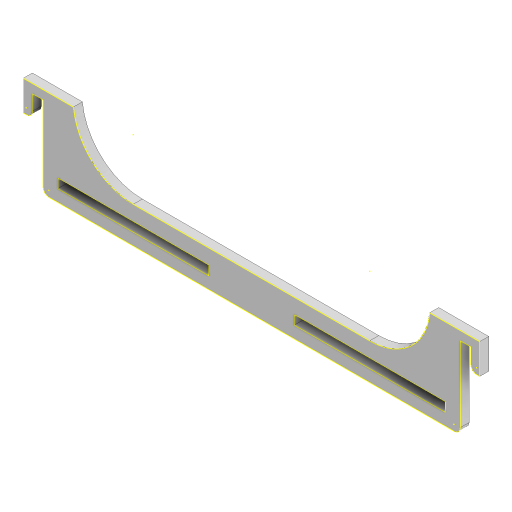
# Autodesk Inventor part: side
Saved by Autodesk Inventor 2023 (Build 270158000, 158)
## iProperties
Created: 2022-05-18
Part Number: side
Material: Generic
Document SubType Name: Modeling
Designer: Thomas
Density: 1 g/cm^3
Appearance: Default
Author: Thomas
Autodesk Inventor part; units mm, degrees
ref_plane "YZ Plane" through (0, 0, 0) normal (1, 0, 0) x (0, 1, 0)
ref_plane "XZ Plane" through (0, 0, 0) normal (0, 1, 0) x (-1, 0, 0)
ref_plane "XY Plane" through (0, 0, 0) normal (0, 0, 1) x (1, 0, 0)
sketch "Sketch1" plane through (0, 0, 0) normal (0, 0, 1) x (1, 0, 0)
  line L0 (0, 0) -> (138.5, 0)
  line L1 (138.5, 0) -> (138.5, -28)
  line L2 (136.5, -30) -> (2, -30)
  line L3 (0, -28) -> (0, 0)
  line L4 (0, 0) -> (-3.5, 0)
  line L5 (-3.5, 0) -> (-3.5, -3)
  line L6 (-3.5, -3) -> (0, -3)
  line L7 (0, -3) -> (0, 0)
  line L8 (-3.5, 0) -> (-6.5, 0)
  line L9 (-6.5, 0) -> (-6.5, -10)
  line L10 (-6.5, -10) -> (-5.5, -10)
  line L11 (-3.5, -8) -> (-3.5, 0)
  line L12 (138.5, -3) -> (142, -3)
  line L13 (142, -3) -> (142, 0)
  line L14 (142, 0) -> (138.5, 0)
  line L15 (138.5, 0) -> (138.5, -3)
  line L16 (142, 0) -> (145, 0)
  line L17 (145, 0) -> (145, -10)
  line L18 (145, -10) -> (144, -10)
  line L19 (142, -8) -> (142, 0)
  arc A0 (-5.5, -10) -> (-3.5, -8) centre (-5.5, -8) ccw
  arc A1 (142, -8) -> (144, -10) centre (144, -8) ccw
  line L20 (5, -23) -> (55, -23)
  line L21 (55, -23) -> (55, -26)
  line L22 (55, -26) -> (5, -26)
  line L23 (5, -26) -> (5, -23)
  line L24 (83.5, -23) -> (133.5, -23)
  line L25 (133.5, -23) -> (133.5, -26)
  line L26 (133.5, -26) -> (83.5, -26)
  line L27 (83.5, -26) -> (83.5, -23)
  arc A2 (0, -28) -> (2, -30) centre (2, -28) ccw
  arc A3 (136.5, -30) -> (138.5, -28) centre (136.5, -28) ccw
  point P0 (138.5, -30)
  point P1 (0, -30)
  point P2 (-3.5, -10)
  point P3 (142, -10)
  dimension "d0" = 138.5
  dimension "d1" = 30
  dimension "d2" = 3.5
  dimension "d3" = 3
  dimension "d4" = 3
  dimension "d5" = 10
  dimension "d6" = 3.5
  dimension "d7" = 3
  dimension "d8" = 3
  dimension "d9" = 10
  dimension "d10" = 2
  dimension "d11" = 3
  dimension "d12" = 20
  dimension "d13" = 5
  dimension "d14" = 50
  dimension "d15" = 3
  dimension "d16" = 5
  dimension "d17" = 50
  dimension "d18" = 2
  constraints: 56 end point, 14 parallel, 9 point on line, 8 point on circle, 8 tangent, 7 horizontal, 7 perpendicular, 4 centre point, 2 collinear, 2 equal radius
  measures "d0" distance of point (138.5, -30) point (0, -30)
  measures "d1" distance of L0.end point (138.5, -30)
  measures "d2" distance of L6.end L5.end
  measures "d3" distance of L5.end L4.end
  measures "d4" distance of point (-3.5, -10) L9.end
  measures "d5" distance of L9.end L8.end
  measures "d6" distance of L14.end L13.end
  measures "d7" distance of L13.end L12.end
  measures "d8" distance of L17.end point (142, -10)
  measures "d9" distance of L16.end L17.end
  measures "d10" radius of A0
  measures "d11" distance of L22.end L20.start
  measures "d12" distance between parallel lines of L6 L20
  measures "d13" distance between parallel lines of L3 L23
  measures "d14" distance of L20.start L20.end
  measures "d15" distance of L24.end L25.end
  measures "d16" distance between parallel lines of L1 L25
  measures "d17" distance of L24.start L24.end
  measures "d18" radius of A2
extrude "Extrusion1" add sketch "Sketch1" along normal blind 3
sketch "Sketch2" plane through (0, 0, 3) normal (0, 0, 1) x (1, 0, 0)
  line L0 (145, 0) -> (-6.5, 0) projected
  line L1 (10, 0) -> (128.5, 0)
  line L2 (128.5, 0) -> (128.5, 2)
  line L3 (108.5, -18) -> (30, -18)
  line L4 (10, 2) -> (10, 0)
  line L5 (5, -23) -> (55, -23) projected
  line L6 (0, -3) -> (0, -28) projected
  line L7 (138.5, -28) -> (138.5, -3) projected
  arc A0 (10, 2) -> (30, -18) centre (30, 2) ccw
  arc A1 (108.5, -18) -> (128.5, 2) centre (108.5, 2) ccw
  point P0 (0, 0)
  point P1 (128.3997, 0)
  point P2 (10.1003, 0)
  dimension "d21" = 5
  dimension "d22" = 10
  dimension "d23" = 10
  dimension "d24" = 20
  constraints: 8 end point, 4 point on circle, 4 tangent, 2 centre point, 2 parallel, 1 equal radius, 1 horizontal, 1 perpendicular, 1 point on line
  measures "d21" distance between parallel lines of L3 L5
  measures "d22" distance between parallel lines of L4 L6
  measures "d23" distance between parallel lines of L7 L2
  measures "d24" radius of A0
extrude "Extrusion2" cut sketch "Sketch2" against normal blind 10 contours A1 L3 A0 L0
sketch "Sketch3" plane through (0, 0, 3) normal (0, 0, 1) x (1, 0, 0)
  arc A0 (10.1003, 0) -> (30, -18) centre (30, 2) ccw projected
  line L0 (10.1003, 0) -> (-6.5, 0) projected
  line L1 (-6.5, 0) -> (-6.5, -10) projected
  line L2 (-6.5, -10) -> (-5.5, -10) projected
  arc A1 (-5.5, -10) -> (-3.5, -8) centre (-5.5, -8) ccw projected
  line L3 (-3.5, -8) -> (-3.5, -3) projected
  line L4 (-3.5, -3) -> (0, -3) projected
  line L5 (0, -3) -> (0, -28) projected
  arc A2 (0, -28) -> (2, -30) centre (2, -28) ccw projected
  line L6 (2, -30) -> (136.5, -30) projected
  arc A3 (136.5, -30) -> (138.5, -28) centre (136.5, -28) ccw projected
  line L7 (138.5, -28) -> (138.5, -3) projected
  line L8 (138.5, -3) -> (142, -3) projected
  line L9 (142, -3) -> (142, -8) projected
  arc A4 (142, -8) -> (144, -10) centre (144, -8) ccw projected
  line L10 (144, -10) -> (145, -10) projected
  line L11 (145, -10) -> (145, 0) projected
  line L12 (145, 0) -> (128.3997, 0) projected
  arc A5 (108.5, -18) -> (128.3997, 0) centre (108.5, 2) ccw projected
  line L13 (108.5, -18) -> (30, -18) projected
  line L14 (83.5, -23) -> (133.5, -23) projected
  line L15 (133.5, -23) -> (133.5, -26) projected
  line L16 (133.5, -26) -> (83.5, -26) projected
  line L17 (83.5, -26) -> (83.5, -23) projected
  line L18 (5, -23) -> (55, -23) projected
  line L19 (55, -23) -> (55, -26) projected
  line L20 (55, -26) -> (5, -26) projected
  line L21 (5, -26) -> (5, -23) projected
  point P0 (0, 0)
equation "\"d15\" = d11"
equation "\"d16\" = d13"
equation "\"d17\" = d14"
body "Solid1"
